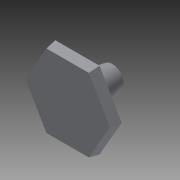
# Autodesk Inventor part: Driven Pin
Saved by Autodesk Inventor 2018 (Build 220112000, 112)
## iProperties
Created: 2018-01-22
Part Number: Driven Pin
Material: Generic
Document SubType Name: Modeling
Designer: Rus
Density: 1 g/cm^3
Appearance: Default
Author: Rus
Autodesk Inventor part; units mm, degrees
note: some values were not read from the file. Chosen so that the rebuilt part matches the saved one: second side of "Extrusion1".
ref_plane "YZ Plane" through (0, 0, 0) normal (1, 0, 0) x (0, 1, 0)
ref_plane "XZ Plane" through (0, 0, 0) normal (0, 1, 0) x (-1, 0, 0)
ref_plane "XY Plane" through (0, 0, 0) normal (0, 0, 1) x (1, 0, 0)
sketch "Sketch1" plane through (0, 0, 0) normal (0, 0, 1) x (1, 0, 0)
  circle A0 centre (0, 0) radius 5.644444
  dimension "d0" = 11.28889
  constraints: 1 centre point, 1 coincident
  measures "d0" diameter of A0
extrude "Extrusion1" add sketch "Sketch1" against normal blind 11.288889 draft -10
sketch "Sketch3" plane through (0, 0, 0) normal (0, 0, 1) x (1, 0, 0)
  circle A0 centre (0, 0) radius 3.653909
  line L0 (-14.2875, 0) -> (-7.14375, 12.373338)
  line L1 (-7.14375, 12.373338) -> (7.14375, 12.373338)
  line L2 (7.14375, 12.373338) -> (14.2875, 0)
  line L3 (14.2875, 0) -> (7.14375, -12.373338)
  line L4 (7.14375, -12.373338) -> (-7.14375, -12.373338)
  line L5 (-7.14375, -12.373338) -> (-14.2875, 0)
  line L6 (0, 0) -> (-14.2875, 0) construction
  dimension "d11" = 28.575
  constraints: 14 end point, 1 coincident, 1 horizontal, 13 other
  measures "d11" distance of L0.start L2.end
sketch "Sketch3 outline for Extrusion3" plane through (0, 0, 0) normal (0, 0, 1) x (1, 0, 0)
  line L0 (-14.2875, 0) -> (-7.14375, 12.373338)
  line L1 (-7.14375, 12.373338) -> (7.14375, 12.373338)
  line L2 (7.14375, 12.373338) -> (14.2875, 0)
  line L3 (14.2875, 0) -> (7.14375, -12.373338)
  line L4 (7.14375, -12.373338) -> (-7.14375, -12.373338)
  line L5 (-7.14375, -12.373338) -> (-14.2875, 0)
extrude "Extrusion3" add sketch "Sketch3 outline for Extrusion3" along normal blind 3.175 draft -10
body "Solid1"
